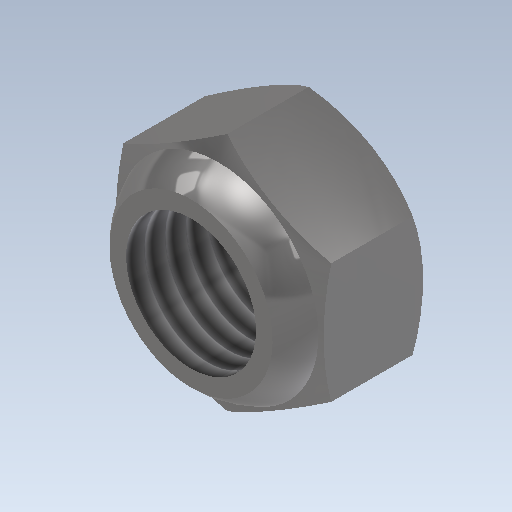
# Autodesk Inventor part: M5 Nylock
Saved by Autodesk Inventor 2020.3 (Build 243373000, 373)
## iProperties
Created: 2016-04-10
Part Number: M5 Nylock
Material: Generic
Document SubType Name: Modeling
Designer: Ben
Density: 1 g/cm^3
Appearance: Default
Mass: 0.1605 g
Surface Area: 2.64502 cm^2
Volume: 0.1605 cm^3
Author: Ben
Autodesk Inventor part; units mm, degrees
ref_plane "YZ Plane" through (0, 0, 0) normal (1, 0, 0) x (0, 1, 0)
ref_plane "XZ Plane" through (0, 0, 0) normal (0, 1, 0) x (-1, 0, 0)
ref_plane "XY Plane" through (0, 0, 0) normal (0, 0, 1) x (1, 0, 0)
sketch "Sketch1" plane through (0, 0, 0) normal (0, 0, 1) x (1, 0, 0)
  line L0 (4, -2.3094) -> (0, -4.6188)
  line L1 (0, -4.6188) -> (-4, -2.3094)
  line L2 (-4, -2.3094) -> (-4, 2.3094)
  line L3 (-4, 2.3094) -> (0, 4.6188)
  line L4 (0, 4.6188) -> (4, 2.3094)
  line L5 (4, 2.3094) -> (4, -2.3094)
  circle A0 centre (0, 0) radius 2.5
  dimension "d0" = 8
  dimension "d1" = 5
  constraints: 12 end point, 2 coincident, 1 centre point, 13 other
  measures "d0" distance between parallel lines of L5 L2
  measures "d1" diameter of A0
extrude "Extrusion1" add sketch "Sketch1" along normal blind 5
sketch "Sketch4" plane through (0, 0, 0) normal (1, 0, 0) x (0, 1, 0)
  line L0 (-4.6188, 0) -> (-2.3094, 0) projected
  line L1 (-4.6188, 0) -> (-4.6188, 5) projected
  line L2 (-2.3094, 5) -> (-4.6188, 5) projected
  line L3 (-2.3094, 0) -> (-2.3094, 5) projected
  line L4 (2.3094, 0) -> (4.6188, 0) projected
  line L5 (2.3094, 0) -> (2.3094, 5) projected
  line L6 (4.6188, 5) -> (2.3094, 5) projected
  line L7 (4.6188, 0) -> (4.6188, 5) projected
  arc A0 (-3.1388, 5) -> (-3.854, 3.9517) centre (-0.7691, 2.615) ccw
  arc A1 (-3.854, 3.9517) -> (-4.6188, 3.6047) centre (-1.2465, -2.8098) ccw
  line L8 (0, 0) -> (0, 9.301) construction
  arc A2 (3.7221, 0) -> (4.6188, 0.5597) centre (0, 6.9619) ccw
  arc A3 (-4.6188, 0.4688) -> (-3.8763, 0) centre (0, 6.9619) ccw
  constraints: 8 point on circle, 7 point on line, 4 centre point, 2 end point, 1 parallel
revolve "Revolution3" cut sketch "Sketch4" angle 360 about axis through (0, 0, 0) along (0, 0, 1) contours L1 A3 L0 | L1 L2 A0 A1
thread "Thread1" size "M5x0.8" class "6H" standard "ANSI Metric M Profile" full length
body "Solid1"
